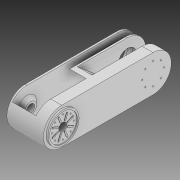
# Autodesk Inventor part: Link1
Saved by Autodesk Inventor 2020 (Build 240168000, 168)
## iProperties
Created: 2021-03-19
Part Number: Link1
Material: Generic
Document SubType Name: Modeling
Designer: DDeGo
Density: 1 g/cm^3
Appearance: Default
Author: DDeGo
Autodesk Inventor part; units mm, degrees
ref_plane "YZ Plane" through (0, 0, 0) normal (1, 0, 0) x (0, 1, 0)
ref_plane "XZ Plane" through (0, 0, 0) normal (0, 1, 0) x (-1, 0, 0)
ref_plane "XY Plane" through (0, 0, 0) normal (0, 0, 1) x (1, 0, 0)
sketch "Sketch1" plane through (0, 0, 0) normal (1, 0, 0) x (0, 1, 0)
  line L0 (0, 0) -> (0, -250) construction
  line L1 (-50, 0) -> (-50, -250)
  line L2 (50, -250) -> (50, 0)
  arc A0 (50, 0) -> (-50, 0) centre (0, 0) ccw
  arc A1 (-50, -250) -> (50, -250) centre (0, -250) ccw
  circle A2 centre (0, 0) radius 25 construction
  circle A3 centre (0, -250) radius 25
  point P0 (0, -125)
  dimension "d0" = 50
  dimension "d1" = 250
  dimension "d2" = 50
  constraints: 8 end point, 4 centre point, 4 point on circle, 4 tangent, 2 coincident, 1 equal radius, 1 midpoint, 1 parallel, 1 vertical
  measures "d0" radius of A0
  measures "d1" distance of L0.start L0.end
  measures "d2" diameter of A2
extrude "Extrusion1" add sketch "Sketch1" along normal blind 100
sketch "Sketch2" plane through (0, 50, 0) normal (0, 1, 0) x (1, 0, 0)
  line L0 (70, 195) -> (30, 195)
  line L1 (30, 195) -> (30, 305)
  line L2 (30, 305) -> (70, 305)
  line L3 (70, 305) -> (70, 195)
  line L4 (0, 250) -> (100, 250) construction
  line L5 (70, 195) -> (30, 305) construction
  line L6 (30, 195) -> (70, 305) construction
  line L7 (0, 300) -> (100, 300) construction
  line L8 (0, 250) -> (0, 300) projected
  line L9 (100, 250) -> (100, 300) projected
  point P0 (0, 0)
  point P1 (50, 250)
  dimension "d5" = 5
  dimension "d24" = 30
  dimension "d25" = 30
  constraints: 12 end point, 3 midpoint, 2 parallel, 1 horizontal, 1 perpendicular
  measures "d5" distance between parallel lines of L2 L7
  measures "d24" distance between parallel lines of L8 L1
  measures "d25" distance between parallel lines of L9 L3
extrude "Extrusion2" cut sketch "Sketch2" against normal through all
sketch "Sketch3" plane through (70, 50, -250) normal (-1, 0, 0) x (0, 0, 1)
  line L0 (-170.3451, -192.9365) -> (170.3451, 92.9365) construction
  circle A0 centre (0, -50) radius 25 projected
  line L1 (-138.2057, -231.2388) -> (202.4845, 54.6343)
  line L2 (138.2057, 131.2388) -> (-202.4845, -154.6343)
  arc A1 (-202.4845, -154.6343) -> (-138.2057, -231.2388) centre (-170.3451, -192.9365) ccw
  arc A2 (202.4845, 54.6343) -> (138.2057, 131.2388) centre (170.3451, 92.9365) ccw
  arc A3 (0, 0) -> (0, -100) centre (0, -50) ccw projected
  line L3 (0, -50) -> (322.1538, -50) construction
  point P0 (250, -50)
  dimension "d96" = 140
  constraints: 10 end point, 4 point on circle, 4 tangent, 2 centre point, 1 equal radius, 1 horizontal, 1 midpoint, 1 parallel
  measures "d96" angle of L3 L0
extrude "Extrusion3" cut sketch "Sketch3" along normal up to surface (40 mm away)
sketch "Sketch4" plane through (100, 0, 0) normal (1, 0, 0) x (0, 0, -1)
  circle A0 centre (0, 0) radius 42.5
  dimension "d14" = 85
  constraints: 1 centre point, 1 coincident
  measures "d14" diameter of A0
extrude "Extrusion4" add sketch "Sketch4" along normal blind 3
sketch "Sketch5" plane through (103, 0, 0) normal (1, 0, 0) x (0, 0, -1)
  line L0 (0, 0) -> (30, 0) construction
  circle A0 centre (30, 0) radius 1.65
  dimension "d17" = 30
  dimension "d18" = 3.3
  constraints: 2 end point, 1 centre point, 1 coincident, 1 horizontal
  measures "d17" distance of L0.start L0.end
  measures "d18" diameter of A0
extrude "Extrusion5" cut sketch "Sketch5" against normal blind 15
pattern_circular "Circular Pattern1" count 8 over 360 about axis through (100, 0, 0) along (1, 0, 0) of "Extrusion5"
ref_plane "Work Plane1" through (5, 0, 0) normal (-1, 0, 0) x (0, 0, 1)
ref_plane "Work Plane2" through (25, 0, -250) normal (1, 0, 0) x (0, 0, -1)
sketch "Sketch7" plane through (5, 0, 0) normal (-1, 0, 0) x (0, 0, 1)
  arc A0 (0, -50) -> (0, 50) centre (0, 0) ccw projected
  line L0 (-250, 50) -> (0, 50) projected
  arc A1 (-250, 50) -> (-250, -50) centre (-250, 0) ccw projected
  line L1 (0, -50) -> (-250, -50) projected
  circle A2 centre (-250, 0) radius 25 construction
  arc A3 (0, -40) -> (40, 0) centre (0, 0) ccw
  line L2 (0, -40) -> (-250, -40)
  arc A4 (-250, 40) -> (-290, 0) centre (-250, 0) ccw construction
  line L3 (-250, 40) -> (0, 40) construction
  line L4 (40, 0) -> (40, 114.8918)
  line L5 (40, 114.8918) -> (-290, 114.8918)
  line L6 (-290, 114.8918) -> (-290, 0)
  arc A5 (40, 0) -> (0, 40) centre (0, 0) ccw construction
  arc A6 (-290, 0) -> (-250, -40) centre (-250, 0) ccw
  point P0 (-290, 30)
  point P1 (40, 30)
  dimension "d31" = 10
  dimension "d32" = 10
  dimension "d33" = 10
  constraints: 10 end point, 8 point on circle, 4 centre point, 2 vertical, 1 perpendicular
  measures "d31" distance between parallel lines of L1 L2
  measures "d32" radial gap between concentric circles of A0 A3
  measures "d33" radial gap between concentric circles of A1 A6
extrude "Extrusion6" cut sketch "Sketch7" against normal up to surface (20 mm away) contours L4 A3 L2 A6 L6 A1 L0 A0
sketch "Sketch8" plane through (25, 0, -290) normal (-1, 0, 0) x (0, 0, 1)
  circle A0 centre (40, 0) radius 25 projected
  line L0 (40, 50) -> (290, 50) projected
  arc A1 (40, 50) -> (0, 30) centre (40, 0) ccw projected
  line L1 (0, 30) -> (0, 0) projected
  arc A2 (0, 0) -> (40, -40) centre (40, 0) ccw projected
  line L2 (40, -40) -> (290, -40) projected
  arc A3 (290, -40) -> (330, 0) centre (290, 0) ccw projected
  line L3 (330, 0) -> (330, 30) projected
  arc A4 (330, 30) -> (290, 50) centre (290, 0) ccw projected
  line L4 (95, -19.1199) -> (95, -50) projected
  line L5 (95, -19.1199) -> (95, -50) projected
  line L6 (40, 50) -> (290, 50) projected
  line L7 (192.9311, 50) -> (95, -32.174)
  line L8 (95, -19.1199) -> (177.3739, 50) projected
  point P0 (95, -32.174)
  point P1 (95, -40)
  point P2 (103.5899, -40)
  dimension "d97" = 10
  constraints: 2 end point, 2 point on line, 1 parallel
  measures "d97" distance between parallel lines of L7 L8
extrude "Extrusion7" cut sketch "Sketch8" against normal up to surface (45 mm away) contours A0 | L0 A4 L3 A3 L2 L4 L7
sketch "Sketch9" plane through (0, 0, 0) normal (-1, 0, 0) x (0, 0, 1)
  circle A0 centre (0, 0) radius 11.05
  dimension "d40" = 22.1
  constraints: 1 centre point, 1 coincident
  measures "d40" diameter of A0
extrude "Extrusion8" cut sketch "Sketch9" against normal up to surface (5 mm away)
sketch "Sketch10" plane through (5, 0, 0) normal (1, 0, 0) x (0, 0, -1)
  circle A0 centre (0, 0) radius 11.05 projected
  circle A1 centre (0, 0) radius 16.05
  dimension "d43" = 5
  constraints: 1 centre point, 1 coincident
  measures "d43" radial gap between concentric circles of A1 A0
extrude "Extrusion9" add sketch "Sketch10" along normal blind 10
chamfer "Chamfer1" distance 10 angle 45 1 edges at (5, 0, 16.05)
sketch "Sketch14" plane through (70, 0, -250) normal (-1, 0, 0) x (0, 0, 1)
  circle A0 centre (0, 0) radius 25 projected
  circle A1 centre (0, 0) radius 47.55
  point P0 (250, 0)
  dimension "d62" = 95.1
  constraints: 1 centre point, 1 coincident
  measures "d62" diameter of A1
extrude "Extrusion13" cut sketch "Sketch14" against normal blind 10
sketch "Sketch15" plane through (80, 0, -250) normal (-1, 0, 0) x (0, 0, 1)
  circle A0 centre (0, 0) radius 25 projected
  circle A1 centre (0, 0) radius 44.55
  circle A2 centre (0, 0) radius 47.55 projected
  point P0 (250, 0)
  dimension "d65" = 3
  constraints: 1 centre point, 1 coincident
  measures "d65" radial gap between concentric circles of A2 A1
extrude "Extrusion14" cut sketch "Sketch15" against normal blind 0.5 contours A1
sketch "Sketch16" plane through (80.5, 0, -250) normal (-1, 0, 0) x (0, 0, 1)
  circle A0 centre (0, 0) radius 25 projected
  circle A1 centre (0, 0) radius 40
  point P0 (250, 0)
  dimension "d68" = 80
  constraints: 1 centre point, 1 coincident
  measures "d68" diameter of A1
extrude "Extrusion15" cut sketch "Sketch16" against normal blind 15.5
sketch "Sketch17" plane through (100, 0, 0) normal (1, 0, 0) x (0, 0, -1)
  circle A0 centre (250, 0) radius 25 construction
  circle A1 centre (250, 0) radius 30 construction
  circle A2 centre (250, 30) radius 1.6
  circle A3 centre (228.7868, 21.2132) radius 1.6
  circle A4 centre (220, 0) radius 1.6
  circle A5 centre (228.7868, -21.2132) radius 1.6
  circle A6 centre (250, -30) radius 1.6
  circle A7 centre (271.2132, -21.2132) radius 1.6
  circle A8 centre (280, 0) radius 1.6
  circle A9 centre (271.2132, 21.2132) radius 1.6
  point P0 (0, 0)
  dimension "d71" = 60
  dimension "d72" = 3.2
  dimension "d75" = 360
  constraints: 8 centre point, 2 vertical alignment, 1 coincident, 19 other
  measures "d72" diameter of A2
extrude "Extrusion16" cut sketch "Sketch17" against normal blind 15.5
sketch "Sketch18" plane through (100, 0, 0) normal (1, 0, 0) x (0, 0, -1)
  circle A0 centre (250, 0) radius 25 projected
  point P0 (0, 0)
extrude "Extrusion17" add sketch "Sketch18" against normal up to surface (4 mm away)
sketch "Sketch19" plane through (103, 0, 0) normal (1, 0, 0) x (0, 0, -1)
  circle A0 centre (0, 0) radius 11.05
  dimension "d81" = 22.1
  constraints: 1 centre point, 1 coincident
  measures "d81" diameter of A0
extrude "Extrusion18" cut sketch "Sketch19" against normal through all
sketch "Sketch20" plane through (103, 0, 0) normal (1, 0, 0) x (0, 0, -1)
  circle A0 centre (0, 0) radius 38
  circle A1 centre (0, 0) radius 42.5 projected
  dimension "d84" = 76
  constraints: 1 centre point, 1 coincident
  measures "d84" diameter of A0
extrude "Extrusion19" add sketch "Sketch20" along normal blind 2
sketch "Sketch21" plane through (103, 0, 0) normal (1, 0, 0) x (0, 0, -1)
  line L0 (0, 0) -> (-8.6104, 20.7873) construction
  circle A0 centre (-21.2132, 21.2132) radius 1.65 projected
  line L1 (-8.6104, 20.7873) -> (-21.2132, 21.2132) construction
  circle A1 centre (0, 30) radius 1.65 projected
  line L2 (-8.6104, 20.7873) -> (0, 30) construction
  line L3 (-11.4805, 27.7164) -> (-5.7403, 13.8582) construction
  line L4 (-13.3283, 26.951) -> (-7.588, 13.0928)
  line L5 (-3.8925, 14.6236) -> (-9.6327, 28.4818)
  arc A2 (-9.6327, 28.4818) -> (-13.3283, 26.951) centre (-11.4805, 27.7164) ccw
  arc A3 (-7.588, 13.0928) -> (-3.8925, 14.6236) centre (-5.7403, 13.8582) ccw
  dimension "d87" = 15
  dimension "d88" = 2
  dimension "d89" = 22.5
  constraints: 14 end point, 4 point on circle, 4 tangent, 2 centre point, 1 equal length, 1 midpoint, 1 parallel, 1 point on line
  measures "d87" distance of L3.start L3.end
  measures "d88" radius of A2
  measures "d89" distance of L0.start L0.end
extrude "Extrusion20" add sketch "Sketch21" along normal blind 0.8 contours A2 L5 A3 L4
fillet "Fillet2" radius 0.2 4 edges at (103.8, 21.5527, 6.7626) (103.8, 29.5641, 12.2459) (103.8, 20.0219, 10.4581) (103.8, 12.0104, 4.9749)
pattern_circular "Circular Pattern2" count 8 over 360 about axis through (103, 0, 0) along (-1, 0, 0) of "Extrusion20", "Fillet2"
equation "\"d32\" = d31"
equation "\"d33\" = d31"
body "Solid1"
